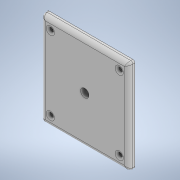
# Autodesk Inventor part: engine_lid
Saved by Autodesk Inventor 2020.1 (Build 241239000, 239)
## iProperties
Created: 2022-02-13
Part Number: engine_lid
Material: Generic
Document SubType Name: Modeling
Designer: OEM
Density: 1 g/cm^3
Appearance: Default
Author: OEM
Autodesk Inventor part; units mm, degrees
ref_plane "YZ Plane" through (0, 0, 0) normal (1, 0, 0) x (0, 1, 0)
ref_plane "XZ Plane" through (0, 0, 0) normal (0, 1, 0) x (-1, 0, 0)
ref_plane "XY Plane" through (0, 0, 0) normal (0, 0, 1) x (1, 0, 0)
sketch "Sketch1" plane through (0, 0, 0) normal (0, 0, 1) x (1, 0, 0)
  circle A0 centre (0, 0) radius 18.5
  line L0 (-21, 22.5) -> (21, 22.5)
  line L1 (21, 22.5) -> (21, -22.5)
  line L2 (21, -22.5) -> (-21, -22.5)
  line L3 (-21, -22.5) -> (-21, 22.5)
  line L4 (-38, 0) -> (59, 0) construction
  line L5 (0, 34) -> (0, -33) construction
  line L6 (-21, -22.5) -> (21, 22.5) construction
  line L7 (21, -22.5) -> (-21, 22.5) construction
  circle A1 centre (16.5, 17.6786) radius 1
  circle A2 centre (-16.5, 17.6786) radius 1
  circle A3 centre (16.5, -17.6786) radius 1
  circle A4 centre (-16.5, -17.6786) radius 1
  circle A5 centre (0, 0) radius 2
  dimension "d1" = 37
  dimension "d2" = 42
  dimension "d3" = 45
  dimension "d4" = 21
  dimension "d5" = 22.5
  dimension "d6" = 2
  dimension "d7" = 4.5
  dimension "d8" = 4
  constraints: 16 end point, 6 centre point, 3 point on line, 3 symmetric about line, 2 horizontal, 2 parallel, 1 coincident, 1 perpendicular, 1 vertical, 3 other
  measures "d1" diameter of A0
  measures "d2" distance of L1.end L2.end
  measures "d3" distance of L0.end L1.end
  measures "d4" distance between parallel lines of L5 L1
  measures "d5" distance between parallel lines of L0 L4
  measures "d6" diameter of A1
  measures "d7" distance from line of L1 A1.centre
  measures "d8" diameter of A5
extrude "Extrusion1" add sketch "Sketch1" along normal blind 3 contours L0 L1 L2 L3
extrude "Extrusion2" add sketch "Sketch1" along normal blind 3 and the other way blind 2 contours A0
fillet "Fillet1" radius 1 4 edges at (15.5, 17.6786, 3) (-17.5, 17.6786, 3) (-17.5, -17.6786, 3) (15.5, -17.6786, 3)
fillet "Fillet2" radius 2 4 edges at (0, 22.5, 3) (21, 0, 3) (0, -22.5, 3) (-21, 0, 3)
fillet "Fillet3" radius 1 8 edges at (-20.4142, 21.9142, 2.4142) (-21, 22.5, 0.5) (20.4142, 21.9142, 2.4142) (21, 22.5, 0.5) (21, -22.5, 0.5) (20.4142, -21.9142, 2.4142) (-20.4142, -21.9142, 2.4142) (-21, -22.5, 0.5)
equation "\"d4\" = 0.5 * d2"
equation "\"d5\" = 0.5 * d3"
body "Solid1"
